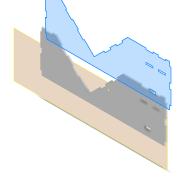
# Autodesk Inventor part: Frontal
Saved by Autodesk Inventor 2022 (Build 260153000, 153)
## iProperties
Created: 2022-06-06
Part Number: Frontal
Material: Generic
Document SubType Name: Modeling
Designer: ADMIN
Density: 1 g/cm^3
Appearance: Default
Author: ADMIN
Autodesk Inventor part; units mm, degrees
ref_plane "YZ Plane" through (0, 0, 0) normal (1, 0, 0) x (0, 1, 0)
ref_plane "XZ Plane" through (0, 0, 0) normal (0, 1, 0) x (-1, 0, 0)
ref_plane "XY Plane" through (0, 0, 0) normal (0, 0, 1) x (1, 0, 0)
ref_plane "Work Plane1" through (-2209.9027, -145.7269, 0) normal (0, 0, 1) x (1, 0, 0)
sketch "Sketch1" plane through (-2209.9027, -145.7269, 0) normal (0, 0, 1) x (1, 0, 0)
  line L0 (1984.9027, 125.3224) -> (1984.9027, 70.7269) projected
  line L1 (1984.9027, 70.7269) -> (2394.9027, 70.7269) projected
  line L2 (2394.9027, 70.7269) -> (2394.9027, 125.3224) projected
  line L3 (2394.9027, 125.3224) -> (2409.9027, 125.3224) projected
  line L4 (2409.9027, 125.3224) -> (2409.9027, 220.7269) projected
  line L5 (2409.9027, 220.7269) -> (2394.9027, 220.7269) projected
  line L6 (1969.9027, 220.7269) -> (1969.9027, 125.3224) projected
  line L7 (1969.9027, 125.3224) -> (1984.9027, 125.3224) projected
  line L8 (1969.9027, 155.7269) -> (1969.9027, 205.7269) projected
  line L9 (1969.9027, 205.7269) -> (1964.9027, 205.7269) projected
  line L10 (1964.9027, 155.7269) -> (1964.9027, 205.7269) projected
  line L11 (1969.9027, 155.7269) -> (1964.9027, 155.7269) projected
  line L12 (1969.9027, 85.7269) -> (1969.9027, 135.7269) projected
  line L13 (1969.9027, 135.7269) -> (1964.9027, 135.7269) projected
  line L14 (1964.9027, 85.7269) -> (1964.9027, 135.7269) projected
  line L15 (1969.9027, 85.7269) -> (1964.9027, 85.7269) projected
  line L16 (1964.9027, 155.7269) -> (1969.9027, 155.7269)
  line L17 (1969.9027, 155.7269) -> (1969.9027, 135.7269)
  line L18 (1969.9027, 135.7269) -> (1964.9027, 135.7269)
  line L19 (1964.9027, 135.7269) -> (1964.9027, 155.7269)
  line L20 (1991.136, 206.6179) -> (1964.9027, 206.6179)
  line L21 (1964.9027, 206.6179) -> (1964.9027, 205.7269)
  line L22 (1964.9027, 205.7269) -> (1991.136, 205.7269)
  line L23 (1991.136, 205.7269) -> (1991.136, 206.6179)
  line L24 (1964.9027, 85.7269) -> (1991.136, 85.7269)
  line L25 (1991.136, 85.7269) -> (1991.136, 70.7269)
  line L26 (1991.136, 70.7269) -> (1964.9027, 70.7269)
  line L27 (1964.9027, 70.7269) -> (1964.9027, 85.7269)
  line L28 (1984.9027, 70.7269) -> (1969.9027, 70.7269)
  line L29 (1969.9027, 70.7269) -> (1969.9027, 125.3224)
  line L30 (1969.9027, 125.3224) -> (1984.9027, 125.3224)
  line L31 (1984.9027, 125.3224) -> (1984.9027, 70.7269)
  line L32 (2414.9027, 155.7269) -> (2414.9027, 205.7269) projected
  line L33 (2414.9027, 205.7269) -> (2409.9027, 205.7269) projected
  line L34 (2409.9027, 155.7269) -> (2409.9027, 205.7269) projected
  line L35 (2414.9027, 155.7269) -> (2409.9027, 155.7269) projected
  line L36 (2414.9027, 85.7269) -> (2414.9027, 135.7269) projected
  line L37 (2414.9027, 135.7269) -> (2409.9027, 135.7269) projected
  line L38 (2409.9027, 85.7269) -> (2409.9027, 135.7269) projected
  line L39 (2414.9027, 85.7269) -> (2409.9027, 85.7269) projected
  line L40 (2409.9027, 70.7269) -> (2394.9027, 70.7269)
  line L41 (2394.9027, 70.7269) -> (2394.9027, 125.3224)
  line L42 (2394.9027, 125.3224) -> (2409.9027, 125.3224)
  line L43 (2409.9027, 125.3224) -> (2409.9027, 70.7269)
  line L44 (2259.9027, 220.7269) -> (2238.8976, 199.7218) projected
  line L45 (2139.9027, 100.7269) -> (2104.5473, 136.0822) projected
  line L46 (2019.9027, 220.7269) -> (2007.4027, 220.7269) projected
  line L47 (2178.7935, 132.5467) -> (2175.258, 136.0822) projected
  line L48 (2104.5473, 136.0822) -> (2101.0118, 132.5467) projected
  line L49 (2101.0118, 132.5467) -> (2079.7986, 153.7599) projected
  line L50 (2079.7986, 153.7599) -> (2083.3341, 157.2954) projected
  line L51 (2083.3341, 157.2954) -> (2062.1209, 178.5086) projected
  line L52 (2062.1209, 178.5086) -> (2058.5854, 174.9731) projected
  line L53 (2058.5854, 174.9731) -> (2037.3722, 196.1863) projected
  line L54 (2037.3722, 196.1863) -> (2040.9077, 199.7218) projected
  line L55 (2238.8976, 199.7218) -> (2242.4332, 196.1863) projected
  line L56 (2242.4332, 196.1863) -> (2221.22, 174.9731) projected
  line L57 (2221.22, 174.9731) -> (2217.6844, 178.5086) projected
  line L58 (2217.6844, 178.5086) -> (2196.4712, 157.2954) projected
  line L59 (2196.4712, 157.2954) -> (2200.0068, 153.7599) projected
  line L60 (2200.0068, 153.7599) -> (2178.7935, 132.5467) projected
  line L61 (2369.9027, 215.7269) -> (2369.9027, 220.7269) projected
  line L62 (2369.9027, 220.7269) -> (2349.9027, 220.7269) projected
  line L63 (2349.9027, 220.7269) -> (2349.9027, 215.7269) projected
  line L64 (2349.9027, 215.7269) -> (2324.9027, 215.7269) projected
  line L65 (2324.9027, 215.7269) -> (2324.9027, 220.7269) projected
  line L66 (2007.4027, 220.7269) -> (2007.4027, 215.7269) projected
  line L67 (2007.4027, 215.7269) -> (1982.4027, 215.7269) projected
  line L68 (1982.4027, 215.7269) -> (1982.4027, 220.7269) projected
  line L69 (2394.9027, 220.7269) -> (2394.9027, 215.7269) projected
  line L70 (2394.9027, 215.7269) -> (2369.9027, 215.7269) projected
  line L71 (2324.9027, 220.7269) -> (2259.9027, 220.7269) projected
  line L72 (2175.258, 136.0822) -> (2139.9027, 100.7269) projected
  line L73 (2040.9077, 199.7218) -> (2019.9027, 220.7269) projected
  line L74 (1982.4027, 220.7269) -> (1969.9027, 220.7269) projected
  point P0 (2209.9027, 145.7269)
  point P1 (1991.136, 21.6179)
  point P2 (1991.136, 6.6179)
  point P3 (1969.9027, 85.7269)
  point P4 (820.3787, 21.6179)
  point P5 (1320.3787, 21.6179)
  point P6 (820.3787, 20.4045)
  point P7 (1984.9027, 70.7269)
  point P8 (1305.3787, -34.1911)
  point P9 (820.3787, 21.6179)
  point P10 (2409.9027, 125.3224)
  point P11 (2394.9027, 70.7269)
  point P12 (1969.9027, 206.6179)
  constraints: 40 end point, 10 parallel, 5 horizontal, 5 perpendicular, 1 collinear, 1 point on line
extrude "Extrusion1" add sketch "Sketch1" along normal blind 5 contours L7 L6 L22 L23 L20 L74 L68 L67 L66 L46 L73 L54 L53 L52 L51 L50 L49 L48 L45 L72 L47 L60 L59 L58 L57 L56 L55 L44 L71 L65 L64 L63 L62 L61 L70 L69 L5 L4 L3 L2 L1 L25 L24 L0 | L0 L24 L12 L7 | L24 L25 L1 L0 | L0 L26 L29 L24 | L12 L15 L14 L13 L6 | L11 L10 L9 L6 | L2 L3 L38 L43 L40 | L6 L20 L23 L22 | L4 L37 L36 L39 L38 | L4 L33 L32 L35
sketch "Sketch3" plane through (-2209.9027, -145.7269, 5) normal (0, 0, 1) x (1, 0, 0)
  point P0 (2209.9027, 145.7269)
sketch "Sketch4" plane through (-2209.9027, -145.7269, 5) normal (0, 0, 1) x (1, 0, 0)
  line L0 (2324.9027, 175.7269) -> (2349.9027, 175.7269)
  line L1 (2349.9027, 175.7269) -> (2349.9027, 170.7269)
  line L2 (2349.9027, 170.7269) -> (2324.9027, 170.7269)
  line L3 (2324.9027, 170.7269) -> (2324.9027, 175.7269)
  line L4 (1969.9027, 220.7269) -> (1969.9027, 205.7269) projected
  line L5 (1969.9027, 155.7269) -> (1969.9027, 135.7269) projected
  line L6 (1969.9027, 135.7269) -> (1964.9027, 135.7269) projected
  line L7 (1964.9027, 135.7269) -> (1964.9027, 85.7269) projected
  line L8 (1969.9027, 70.7269) -> (2409.9027, 70.7269) projected
  line L9 (2409.9027, 85.7269) -> (2414.9027, 85.7269) projected
  line L10 (2414.9027, 85.7269) -> (2414.9027, 135.7269) projected
  line L11 (2414.9027, 135.7269) -> (2409.9027, 135.7269) projected
  line L12 (2409.9027, 135.7269) -> (2409.9027, 155.7269) projected
  line L13 (2409.9027, 155.7269) -> (2414.9027, 155.7269) projected
  line L14 (2414.9027, 155.7269) -> (2414.9027, 205.7269) projected
  line L15 (2414.9027, 205.7269) -> (2409.9027, 205.7269) projected
  line L16 (2409.9027, 205.7269) -> (2409.9027, 220.7269) projected
  line L17 (2409.9027, 220.7269) -> (2394.9027, 220.7269) projected
  line L18 (2369.9027, 175.7269) -> (2394.9027, 175.7269)
  line L19 (2394.9027, 175.7269) -> (2394.9027, 170.7269)
  line L20 (2394.9027, 170.7269) -> (2369.9027, 170.7269)
  line L21 (2369.9027, 170.7269) -> (2369.9027, 175.7269)
  line L22 (2259.9027, 220.7269) -> (2238.8976, 199.7218) projected
  line L23 (2139.9027, 100.7269) -> (2104.5473, 136.0822) projected
  line L24 (2019.9027, 220.7269) -> (2007.4027, 220.7269) projected
  line L25 (1964.9027, 85.7269) -> (1969.9027, 85.7269) projected
  line L26 (2409.9027, 70.7269) -> (2409.9027, 85.7269) projected
  line L27 (1969.9027, 85.7269) -> (1969.9027, 70.7269) projected
  line L28 (1964.9027, 205.7269) -> (1964.9027, 155.7269) projected
  line L29 (1964.9027, 155.7269) -> (1969.9027, 155.7269) projected
  line L30 (2238.8976, 199.7218) -> (2242.4332, 196.1863) projected
  line L31 (2242.4332, 196.1863) -> (2221.22, 174.9731) projected
  line L32 (2221.22, 174.9731) -> (2217.6844, 178.5086) projected
  line L33 (2217.6844, 178.5086) -> (2196.4712, 157.2954) projected
  line L34 (2196.4712, 157.2954) -> (2200.0068, 153.7599) projected
  line L35 (2200.0068, 153.7599) -> (2178.7935, 132.5467) projected
  line L36 (2178.7935, 132.5467) -> (2175.258, 136.0822) projected
  line L37 (2104.5473, 136.0822) -> (2101.0118, 132.5467) projected
  line L38 (2101.0118, 132.5467) -> (2079.7986, 153.7599) projected
  line L39 (2079.7986, 153.7599) -> (2083.3341, 157.2954) projected
  line L40 (2083.3341, 157.2954) -> (2062.1209, 178.5086) projected
  line L41 (2062.1209, 178.5086) -> (2058.5854, 174.9731) projected
  line L42 (2058.5854, 174.9731) -> (2037.3722, 196.1863) projected
  line L43 (2037.3722, 196.1863) -> (2040.9077, 199.7218) projected
  line L44 (2394.9027, 220.7269) -> (2394.9027, 215.7269) projected
  line L45 (2394.9027, 215.7269) -> (2369.9027, 215.7269) projected
  line L46 (2369.9027, 215.7269) -> (2369.9027, 220.7269) projected
  line L47 (2369.9027, 220.7269) -> (2349.9027, 220.7269) projected
  line L48 (2349.9027, 220.7269) -> (2349.9027, 215.7269) projected
  line L49 (2349.9027, 215.7269) -> (2324.9027, 215.7269) projected
  line L50 (2324.9027, 215.7269) -> (2324.9027, 220.7269) projected
  line L51 (2007.4027, 220.7269) -> (2007.4027, 215.7269) projected
  line L52 (2007.4027, 215.7269) -> (1982.4027, 215.7269) projected
  line L53 (1982.4027, 215.7269) -> (1982.4027, 220.7269) projected
  line L54 (2324.9027, 220.7269) -> (2259.9027, 220.7269) projected
  line L55 (2175.258, 136.0822) -> (2139.9027, 100.7269) projected
  line L56 (2040.9077, 199.7218) -> (2019.9027, 220.7269) projected
  line L57 (1982.4027, 220.7269) -> (1969.9027, 220.7269) projected
  line L58 (1969.9027, 205.7269) -> (1964.9027, 205.7269) projected
  point P0 (2209.9027, 145.7269)
  dimension "d16" = 25
  dimension "d17" = 5
  dimension "d18" = 100
  dimension "d19" = 25
  dimension "d20" = 5
  dimension "d22" = 15
  dimension "d25" = 20
  constraints: 16 end point, 4 parallel, 2 horizontal, 2 perpendicular, 1 collinear
  measures "d16" distance of L1.end L2.end
  measures "d17" distance of L0.end L1.end
  measures "d18" distance between parallel lines of L8 L2
  measures "d19" distance of L19.end L20.end
  measures "d20" distance of L18.end L19.end
  measures "d22" distance between parallel lines of L12 L19
  measures "d25" distance between parallel lines of L21 L1
extrude "Extrusion3" cut sketch "Sketch4" against normal blind 5 contours L0 L1 L2 L3 | L18 L19 L20 L21
sketch "Sketch5" plane through (-2209.9027, -145.7269, 5) normal (0, 0, 1) x (1, 0, 0)
  point P0 (2209.9027, 145.7269)
sketch "Sketch6" plane through (-2209.9027, -145.7269, 5) normal (0, 0, 1) x (1, 0, 0)
  line L0 (2394.9027, 175.7269) -> (2394.9027, 170.7269) projected
  line L1 (2394.9027, 170.7269) -> (2369.9027, 170.7269) projected
  line L2 (2369.9027, 170.7269) -> (2369.9027, 175.7269) projected
  line L3 (2369.9027, 175.7269) -> (2394.9027, 175.7269) projected
  line L4 (2349.9027, 175.7269) -> (2349.9027, 170.7269) projected
  line L5 (2349.9027, 170.7269) -> (2324.9027, 170.7269) projected
  line L6 (2324.9027, 170.7269) -> (2324.9027, 175.7269) projected
  line L7 (2324.9027, 175.7269) -> (2349.9027, 175.7269) projected
  line L8 (1964.9027, 85.7269) -> (1969.9027, 85.7269) projected
  line L9 (1969.9027, 85.7269) -> (1969.9027, 70.7269) projected
  line L10 (1969.9027, 70.7269) -> (2409.9027, 70.7269) projected
  line L11 (2409.9027, 70.7269) -> (2409.9027, 85.7269) projected
  line L12 (2409.9027, 85.7269) -> (2414.9027, 85.7269) projected
  line L13 (2414.9027, 85.7269) -> (2414.9027, 135.7269) projected
  line L14 (2414.9027, 135.7269) -> (2409.9027, 135.7269) projected
  line L15 (2409.9027, 135.7269) -> (2409.9027, 155.7269) projected
  line L16 (2409.9027, 155.7269) -> (2414.9027, 155.7269) projected
  line L17 (2414.9027, 155.7269) -> (2414.9027, 205.7269) projected
  line L18 (2414.9027, 205.7269) -> (2409.9027, 205.7269) projected
  line L19 (2409.9027, 205.7269) -> (2409.9027, 220.7269) projected
  line L20 (2409.9027, 220.7269) -> (2394.9027, 220.7269) projected
  line L21 (2394.9027, 220.7269) -> (2394.9027, 215.7269) projected
  line L22 (2394.9027, 215.7269) -> (2369.9027, 215.7269) projected
  line L23 (2369.9027, 215.7269) -> (2369.9027, 220.7269) projected
  line L24 (2369.9027, 220.7269) -> (2349.9027, 220.7269) projected
  line L25 (2349.9027, 220.7269) -> (2349.9027, 215.7269) projected
  line L26 (2349.9027, 215.7269) -> (2324.9027, 215.7269) projected
  line L27 (2324.9027, 215.7269) -> (2324.9027, 220.7269) projected
  line L28 (2259.9027, 220.7269) -> (2238.8976, 199.7218) projected
  line L29 (2238.8976, 199.7218) -> (2242.4332, 196.1863) projected
  line L30 (2242.4332, 196.1863) -> (2221.22, 174.9731) projected
  line L31 (2221.22, 174.9731) -> (2217.6844, 178.5086) projected
  line L32 (2217.6844, 178.5086) -> (2196.4712, 157.2954) projected
  line L33 (2196.4712, 157.2954) -> (2200.0068, 153.7599) projected
  line L34 (2200.0068, 153.7599) -> (2178.7935, 132.5467) projected
  line L35 (2178.7935, 132.5467) -> (2175.258, 136.0822) projected
  line L36 (2139.9027, 100.7269) -> (2104.5473, 136.0822) projected
  line L37 (2104.5473, 136.0822) -> (2101.0118, 132.5467) projected
  line L38 (2101.0118, 132.5467) -> (2079.7986, 153.7599) projected
  line L39 (2079.7986, 153.7599) -> (2083.3341, 157.2954) projected
  line L40 (2083.3341, 157.2954) -> (2062.1209, 178.5086) projected
  line L41 (2062.1209, 178.5086) -> (2058.5854, 174.9731) projected
  line L42 (2058.5854, 174.9731) -> (2037.3722, 196.1863) projected
  line L43 (2037.3722, 196.1863) -> (2040.9077, 199.7218) projected
  line L44 (2019.9027, 220.7269) -> (2007.4027, 220.7269) projected
  line L45 (2007.4027, 220.7269) -> (2007.4027, 215.7269) projected
  line L46 (2007.4027, 215.7269) -> (1982.4027, 215.7269) projected
  line L47 (1982.4027, 215.7269) -> (1982.4027, 220.7269) projected
  line L48 (1969.9027, 220.7269) -> (1969.9027, 205.7269) projected
  line L49 (1964.9027, 205.7269) -> (1964.9027, 155.7269) projected
  line L50 (1964.9027, 155.7269) -> (1969.9027, 155.7269) projected
  line L51 (1969.9027, 155.7269) -> (1969.9027, 135.7269) projected
  line L52 (1969.9027, 135.7269) -> (1964.9027, 135.7269) projected
  line L53 (1964.9027, 135.7269) -> (1964.9027, 85.7269) projected
  line L54 (2339.9027, 100.7269) -> (2359.9027, 100.7269)
  line L55 (2359.9027, 100.7269) -> (2359.9027, 90.7269)
  line L56 (2359.9027, 90.7269) -> (2339.9027, 90.7269)
  line L57 (2339.9027, 90.7269) -> (2339.9027, 100.7269)
  line L58 (2324.9027, 220.7269) -> (2259.9027, 220.7269) projected
  line L59 (2175.258, 136.0822) -> (2139.9027, 100.7269) projected
  line L60 (2040.9077, 199.7218) -> (2019.9027, 220.7269) projected
  line L61 (1982.4027, 220.7269) -> (1969.9027, 220.7269) projected
  line L62 (1969.9027, 205.7269) -> (1964.9027, 205.7269) projected
  point P0 (2209.9027, 145.7269)
  dimension "d26" = 20
  dimension "d27" = 10
  dimension "d28" = 20
  dimension "d29" = 50
  constraints: 8 end point, 2 parallel, 1 horizontal, 1 perpendicular
  measures "d26" distance of L55.end L56.end
  measures "d27" distance of L54.end L55.end
  measures "d28" distance between parallel lines of L10 L56
  measures "d29" distance between parallel lines of L11 L55
extrude "Extrusion4" cut sketch "Sketch6" against normal blind 10 contours L54 L55 L56 L57
equation "\"d19\" = d16"
body "Solid1"
